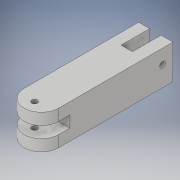
# Autodesk Inventor part: SecondChain
Saved by Autodesk Inventor 2019 (Build 230136000, 136)
## iProperties
Created: 2019-01-18
Part Number: SecondChain
Material: Generic
Document SubType Name: Modeling
Designer: mar22
Density: 1 g/cm^3
Appearance: Default
Author: mar22
Autodesk Inventor part; units mm, degrees
ref_plane "YZ Plane" through (0, 0, 0) normal (1, 0, 0) x (0, 1, 0)
ref_plane "XZ Plane" through (0, 0, 0) normal (0, 1, 0) x (-1, 0, 0)
ref_plane "XY Plane" through (0, 0, 0) normal (0, 0, 1) x (1, 0, 0)
sketch "Sketch1" plane through (0, 0, 0) normal (0, 1, 0) x (-1, 0, 0)
  line L0 (76.2, 0) -> (76.2, -254)
  line L1 (76.2, -254) -> (0, -254)
  line L2 (0, -254) -> (0, 0)
  arc A0 (76.2, 0) -> (0, 0) centre (38.1, 0) ccw
  constraints: 6 end point, 2 point on circle, 1 centre point, 1 parallel
extrude "Extrusion1" add sketch "Sketch1" along normal blind 76.2
sketch "Sketch2" plane through (0, 0, 0) normal (1, 0, 0) x (0, 0, -1)
  line L0 (-38.1, 25.4) -> (25.4, 25.4)
  line L1 (25.4, 25.4) -> (25.4, 50.8)
  line L2 (25.4, 50.8) -> (-38.1, 50.8)
  line L3 (-38.1, 0) -> (-38.1, 76.2) projected
  line L4 (-38.1, 38.1) -> (25.4, 50.8) construction
  line L5 (25.4, 25.4) -> (-38.1, 38.1) construction
  line L6 (-38.1, 50.8) -> (-38.1, 25.4)
  point P0 (0, 0)
  constraints: 12 end point, 2 midpoint, 2 point on line, 1 horizontal, 1 parallel, 1 perpendicular
extrude "Extrusion2" cut sketch "Sketch2" against normal blind 111.125
sketch "Sketch3" plane through (0, 76.2, 0) normal (0, 1, 0) x (1, 0, 0)
  point P0 (0, 0)
  point P1 (-39.0791, -13.8463)
hole "Hole1" at (-39.0791, 76.2, 13.8463) direction (0, -1, 0) diameter 12.7 depth 98.425 tip angle 118
sketch "Sketch5" plane through (0, 0, -254) normal (0, 0, -1) x (-1, 0, 0)
  line L0 (76.2, 0) -> (0, 0) projected
  line L1 (51.7791, 76.2) -> (51.7791, 0)
  line L2 (51.7791, 0) -> (26.3791, 0)
  line L3 (26.3791, 0) -> (26.3791, 76.2)
  line L4 (32.7291, 76.2) -> (45.4291, 76.2) projected
  line L5 (76.2, 76.2) -> (0, 76.2) projected
  line L6 (51.7791, 76.2) -> (24.7587, 76.2)
  point P0 (39.0791, 76.2)
  constraints: 8 end point, 4 point on line, 1 midpoint, 1 parallel
extrude "Extrusion3" cut sketch "Sketch5" against normal blind 63.5
sketch "Sketch6" plane through (0, 0, 0) normal (1, 0, 0) x (0, 0, -1)
  point P0 (0, 0)
  point P1 (230.7386, 44.6045)
hole "Hole2" at (0, 44.6045, -230.7386) direction (-1, 0, 0) diameter 12.7 depth 98.425 tip angle 118
body "Solid1"
